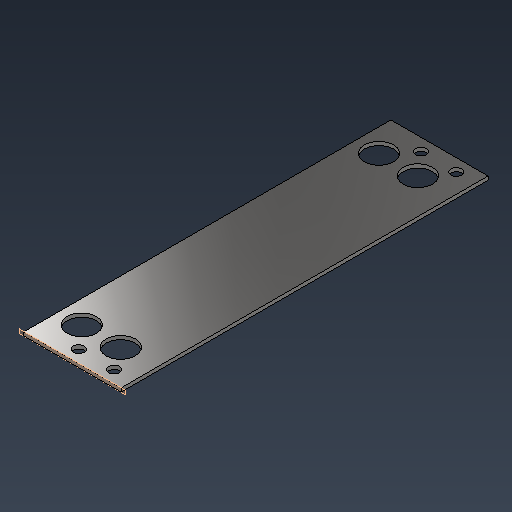
# Autodesk Inventor part: SteelFront
Saved by Autodesk Inventor 2026.2 (Build 302298010, 298A)
## iProperties
Created: 2026-04-07
Part Number: SteelFront
Material: Steel, Alloy
Document SubType Name: Modeling
Designer: szymo
Density: 7.73 g/cm^3
Appearance: Semi-Polished(2)
Mass: 19.6905 g
Surface Area: 54.8833 cm^2
Volume: 2.54729 cm^3
Author: szymo
Autodesk Inventor part; units mm, degrees
ref_plane "YZ Plane" through (0, 0, 0) normal (1, 0, 0) x (0, 1, 0)
ref_plane "XZ Plane" through (0, 0, 0) normal (0, 1, 0) x (-1, 0, 0)
sketch "Sketch1" plane through (0, 0, 0) normal (0, 0, 1) x (1, 0, 0)
  line L0 (0.65, -95.0088) -> (0.65, -83.2008) construction
  line L1 (2.65, -83.2008) -> (2.65, -91.0088) construction
  line L2 (2.65, -91.0088) -> (4.65, -91.0088) construction
  line L3 (4.65, -91.0088) -> (0.65, -95.0088) construction
  circle A0 centre (15.35, -55.1458) radius 14.7 construction
  line L4 (3.0006, -90.8088) -> (30.45, -86.6259)
  line L5 (30.45, -86.6259) -> (30.2994, -85.6374)
  line L6 (30.2994, -85.6374) -> (2.85, -89.8202)
  line L7 (2.85, -89.8202) -> (3.0006, -90.8088)
  line L8 (30.45, -86.6259) -> (30.45, -70.1877) construction
  line L9 (25.65, -86.3458) -> (5.15, -86.3458) projected
  line L10 (5.15, -86.3458) -> (5.15, -69.8458) projected
  line L11 (25.65, -69.8458) -> (5.15, -69.8458) projected
  line L12 (25.65, -86.3458) -> (25.65, -69.8458) projected
  line L13 (0.65, -83.2008) -> (2.65, -83.2008) projected
  dimension "d0" = 1
  dimension "d1" = 0.2
  dimension "d2" = 0.2
  dimension "d3" = 0.4
  dimension "d4" = 0
  dimension "d17" = 27.7662
  constraints: 10 end point, 2 parallel, 1 perpendicular, 1 vertical
  measures "d0" distance between parallel lines of L6 L4
  measures "d1" distance from line of L1 L6.end
  measures "d2" distance from line of L2 L4.start
  measures "d3" distance edge to line of A0 L8
  measures "d4" distance from line of L6 L9.start
  measures "d17" distance of L5.end L6.end
extrude "Extrusion1" [suppressed]
sketch "Sketch2" plane through (30.45, -86.6259, -50) normal (0.1506443, -0.988588, 0) x (0.988588, 0.1506443, 0)
  line L0 (-25.9454, 16.5) -> (-25.9454, 83.5) projected
  line L1 (-27.9685, 0) -> (-27.9685, 3) projected
  circle A0 centre (-5.2783, 96.6469) radius 1.5
  circle A1 centre (-14.8697, 96.6469) radius 1.5
  circle A2 centre (-14.8697, 3.3531) radius 1.5
  circle A3 centre (-5.2783, 3.3531) radius 1.5
  circle A4 centre (-9.5918, 90.5) radius 4
  circle A5 centre (-20.1476, 90.5) radius 4
  circle A6 centre (-9.5918, 9.5) radius 4
  circle A7 centre (-20.1476, 9.5) radius 4
  line L2 (-27.3313, 20) -> (-27.3313, 3) projected
  line L3 (-2.2753, 15.5) -> (-24.9339, 15.5) projected
  line L4 (-13.8886, 7.2533) -> (-16.5988, 7.2533) projected
  line L5 (-27.9685, 20) -> (-27.9685, 80) projected
  line L6 (-2.2753, 3.6302) -> (-2.2753, 0) projected
  arc A8 (-7.1381, 5.9818) -> (-2.2753, 3.6302) centre (-5.2753, 3.6302) ccw projected
  arc A9 (-2.2753, 3.6302) -> (-7.1381, 5.9818) centre (-5.2753, 3.6302) ccw projected
  line L7 (-2.2753, 15.5) -> (-2.2753, 3.6302) projected
  line L8 (-27.3313, 3) -> (-27.9685, 3) projected
  ellipse E0 centre (-20.5244, 90.5) end of major axis (-15.9938, 90.5) minor radius 4.5 (-16.5988, 92.7467) -> (-16.5988, 88.2533) ccw projected
  line L9 (-16.5988, 92.7467) -> (-13.8886, 92.7467) projected
  ellipse E1 centre (-9.963, 90.5) end of major axis (-5.4324, 90.5) minor radius 4.5 (-7.1381, 94.0182) -> (-13.8886, 92.7467) ccw projected
  arc A10 (-2.2753, 96.3698) -> (-7.1381, 94.0182) centre (-5.2753, 96.3698) ccw projected
  line L10 (-2.2753, 96.3698) -> (-2.2753, 100) projected
  line L11 (-2.2753, 100) -> (-27.9685, 100) projected
  line L12 (-27.9685, 97) -> (-27.9685, 100) projected
  line L13 (-27.9685, 97) -> (-27.3313, 97) projected
  line L14 (-27.3313, 97) -> (-27.3313, 80) projected
  line L15 (-27.3313, 80) -> (-27.9685, 80) projected
  ellipse E2 centre (-24.9339, 83.5) end of major axis (-25.9454, 83.5) minor radius 1 (-24.9339, 84.5) -> (-25.9454, 83.5) ccw projected
  line L16 (-2.2753, 84.5) -> (-24.9339, 84.5) projected
  line L17 (-2.2753, 84.5) -> (-2.2753, 96.3698) projected
  arc A11 (-7.1381, 94.0182) -> (-2.2753, 96.3698) centre (-5.2753, 96.3698) ccw projected
  ellipse E3 centre (-9.963, 90.5) end of major axis (-5.4324, 90.5) minor radius 4.5 (-13.8886, 88.2533) -> (-7.1381, 94.0182) ccw projected
  line L18 (-13.8886, 88.2533) -> (-16.5988, 88.2533) projected
  circle A12 centre (-15.2437, 96.3698) radius 3 projected
  ellipse E4 centre (-9.963, 9.5) end of major axis (-5.4324, 9.5) minor radius 4.5 (-13.8886, 7.2533) -> (-7.1381, 5.9818) ccw projected
  ellipse E5 centre (-9.963, 9.5) end of major axis (-5.4324, 9.5) minor radius 4.5 (-7.1381, 5.9818) -> (-13.8886, 11.7467) ccw projected
  circle A13 centre (-15.2437, 3.6302) radius 3 projected
  line L19 (-27.9685, 20) -> (-27.3313, 20) projected
  line L20 (-2.2753, 0) -> (-27.9685, 0) projected
  ellipse E6 centre (-20.5244, 9.5) end of major axis (-15.9938, 9.5) minor radius 4.5 (-16.5988, 11.7467) -> (-16.5988, 7.2533) ccw projected
  line L21 (-16.5988, 11.7467) -> (-13.8886, 11.7467) projected
  ellipse E7 centre (-24.9339, 16.5) end of major axis (-25.9454, 16.5) minor radius 1 (-25.9454, 16.5) -> (-24.9339, 15.5) ccw projected
  point P0 (-17.0528, 50)
  point P1 (-16.268, 7.2533)
  point P2 (-16.3079, 7.2533)
  point P3 (-16.3688, 7.2533)
  point P4 (-16.5217, 7.2533)
  point P5 (-16.5463, 7.2533)
  point P6 (-14.6243, 7.2533)
  point P7 (-17.1998, 7.2533)
  point P8 (-9.892, 13.95)
  point P9 (-28.626, 82.5)
  point P10 (-14.5461, 11.7467)
  dimension "d7" = 3
  dimension "d8" = 3
  dimension "d9" = 3
  dimension "d10" = 3
  dimension "d13" = 8
  dimension "d14" = 8
  dimension "d15" = 8
  dimension "d16" = 8
  constraints: 8 centre point, 11 other
  measures "d7" diameter of A0
  measures "d8" diameter of A1
  measures "d9" diameter of A2
  measures "d10" diameter of A3
  measures "d13" diameter of A4
  measures "d14" diameter of A5
  measures "d15" diameter of A7
  measures "d16" diameter of A6
extrude "Extrusion2" [suppressed]
sketch "Sketch5" plane through (0, 0, 0) normal (0, 1, 0) x (-1, 0, 0)
  line L0 (0, -100) -> (0, 0)
  line L1 (0, 0) -> (-26.4787, 0)
  line L2 (-26.4787, 0) -> (-26.4787, -100)
  line L3 (-26.4787, -100) -> (0, -100)
  circle A0 centre (-6.2585, -9.5) radius 4
  circle A1 centre (-21.2257, -96.6288) radius 1.5
  circle A2 centre (-11.5653, -3.3712) radius 1.5
  circle A3 centre (-16.8722, -90.5) radius 4
  circle A4 centre (-16.8722, -9.5) radius 4
  circle A5 centre (-11.5653, -96.6288) radius 1.5
  circle A6 centre (-21.2257, -3.3712) radius 1.5
  circle A7 centre (-6.2585, -90.5) radius 4
  point P0 (0, 0)
  dimension "d2" = 0.2
  constraints: 8 centre point, 8 end point
extrude "Extrusion5" add sketch "Sketch5" against normal blind 1
equation "\"d14\" = d13"
equation "\"d15\" = d13"
equation "\"d16\" = d13"
body "Solid1"
